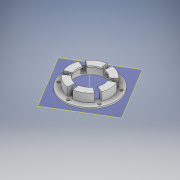
# Autodesk Inventor part: DodatniDržačZaLežaj
Saved by Autodesk Inventor 2020 (Build 240168000, 168)
## iProperties
Created: 2020-10-16
Part Number: DodatniDržačZaLežaj
Material: Generic
Document SubType Name: Modeling
Designer: Sičaja
Density: 1 g/cm^3
Appearance: Default
Author: Sičaja
Autodesk Inventor part; units mm, degrees
ref_plane "YZ Plane" through (0, 0, 0) normal (1, 0, 0) x (0, 1, 0)
ref_plane "XZ Plane" through (0, 0, 0) normal (0, 1, 0) x (-1, 0, 0)
ref_plane "XY Plane" through (0, 0, 0) normal (0, 0, 1) x (1, 0, 0)
sketch "Sketch1" plane through (0, 0, 0) normal (0, 1, 0) x (-1, 0, 0)
  circle A0 centre (0, 0) radius 11.5
  circle A1 centre (0, 0) radius 14.5
  line L0 (13.2396, 5.9129) -> (10.5004, 4.6895)
  line L1 (13.4748, -5.3554) -> (10.6869, -4.2474)
  dimension "d0" = 23
  dimension "d1" = 29
  constraints: 4 end point, 4 point on circle, 2 centre point, 2 coincident
  measures "d0" diameter of A0
  measures "d1" diameter of A1
extrude "Extrusion1" add sketch "Sketch1" along normal blind 6 contours A0 L0 A1 L1 picked at (13.4152, 1.2095)
sketch "Sketch2" plane through (-10.5004, 0, 4.6895) normal (0.4077828, 0, 0.9130789) x (0.9130789, 0, -0.4077828)
  line L0 (-3, 6) -> (0, 6) projected
  line L1 (-3, 6) -> (0.5, 6)
  line L2 (0.5, 6) -> (0.5, 7)
  line L3 (0.5, 7) -> (-3, 7)
  line L4 (-3, 7) -> (-3, 6)
  line L5 (11.5, 8.4) -> (11.5, -1.4) projected
  point P0 (11.5, 0)
  point P1 (0, 6)
  dimension "d4" = 3.5
  dimension "d5" = 1
  constraints: 8 end point, 3 perpendicular, 1 collinear
  measures "d4" distance of L0.start L1.end
  measures "d5" distance of L1.end L2.end
revolve "Revolution1" add sketch "Sketch2" angle 45.74 about axis through (0, 0, 0) along (0, -1, 0)
pattern_circular "Circular Pattern1" count 6 over 360 about axis through (0, 0, 0) along (0, -1, 0) of "Revolution1", "Extrusion1"
ref_plane "Work Plane1" through (1.189, 0, -11.4384) normal (0, -1, 0) x (0.855405, 0, -0.5179597)
sketch "Sketch3" plane through (1.189, 0, -11.4384) normal (0, -1, 0) x (0.855405, 0, -0.5179597)
  circle A0 centre (-6.9417, 9.1686) radius 15.75
  arc A1 (-11.4111, -1.4274) -> (-2.4723, -1.4274) centre (-6.9417, 9.1686) ccw projected
  circle A2 centre (-6.9417, 9.1686) radius 11.5
  point P0 (-2.4723, -1.4274)
  dimension "d10" = 31.5
  constraints: 2 coincident, 1 centre point, 3 other
  measures "d10" diameter of A0
extrude "Extrusion2" add sketch "Sketch3" against normal blind 1
pattern_circular "Circular Pattern2" count 6 over 360 about axis through (0, 0, 0) along (0, -1, 0) of "Extrusion2"
sketch "Sketch6" plane through (1.189, 1, -11.4384) normal (0, 1, 0) x (0.855405, 0, -0.5179597)
  circle A0 centre (-13.5083, -24.5755) radius 1
  point P0 (-6.9417, -9.1686)
  dimension "d22" = 2
  constraints: 1 centre point
  measures "d22" diameter of A0
extrude "Extrusion5" cut sketch "Sketch6" against normal blind 1
sketch "Sketch7" plane through (0, 0, 0) normal (0, -1, 0) x (1, 0, 0)
  circle A0 centre (0, 0) radius 18.5
  circle A1 centre (0, 0) radius 15.75
  dimension "d25" = 37
  constraints: 2 centre point, 1 coincident
  measures "d25" diameter of A0
extrude "Extrusion6" add sketch "Sketch7" against normal blind 1
sketch "Sketch8" plane through (0, 1, 0) normal (0, 1, 0) x (1, 0, 0)
  circle A0 centre (-0.6107, 16.2073) radius 1
  point P0 (0, 0)
  dimension "d28" = 2
  constraints: 1 centre point
  measures "d28" diameter of A0
extrude "Extrusion7" cut sketch "Sketch8" against normal blind 1
pattern_circular "Circular Pattern3" count 6 over 360 about axis through (0, 0, 0) along (0, -1, 0) of "Extrusion7"
sketch "Sketch9" plane through (-10.0439, 6, 4.4856) normal (0.4077828, 0, 0.9130789) x (0.9130789, 0, -0.4077828)
  line L0 (0, 1) -> (-3.5, 1) projected
  line L1 (0, 0) -> (0, 1) projected
  line L2 (-0.5, 0) -> (0, 0) projected
  line L3 (-3.5, -5) -> (-3.5, 1) projected
  line L4 (-3.5, 0) -> (1.5, 0)
  line L5 (1.5, 0) -> (1.5, 1)
  line L6 (1.5, 1) -> (-3.5, 1)
  line L7 (-3.5, 1) -> (-3.5, 0)
  line L8 (11, 2.4) -> (11, -7.4) projected
  point P0 (11, -6)
  dimension "d34" = 5
  dimension "d35" = 1
  constraints: 8 end point, 1 collinear, 1 horizontal, 1 perpendicular, 1 point on line, 1 vertical
  measures "d34" distance of L4.start L4.end
  measures "d35" distance of L4.end L5.end
revolve "Revolution2" add sketch "Sketch9" angle 45.74 about axis through (0, 0, 0) along (0, -1, 0)
pattern_circular "Circular Pattern4" count 6 over 360 about axis through (0, 0, 0) along (0, -1, 0) of "Revolution1", "Revolution2"
body "Solid1"
